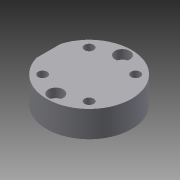
# Autodesk Inventor part: 02-2-0.125-FO1_BM_heads_left-bif
Saved by Autodesk Inventor 2014 SP2 (Build 180246200, 246)
## iProperties
Created: 2020-02-04
Part Number: 02-2-0.125-FO1_BM_heads_left-bif
Material: Generic
Catalog Web Link: www.cadenas.de
Description: FO1 Basic Model Heads_left-Bimba FLAT-1
Vendor: BIMBA
Document SubType Name: Modeling
Designer: psadmin
Manufacturer: BIMBA
Mass: 4.51427 g
Surface Area: 26.3958 cm^2
Volume: 4.51427 cm^3
Density: 1 g/cm^3
Appearance: PSOLRGB-211-211-211
Category: PARTsolutions
Company: BIMBA
Title: 02-2-0.125-FO1_BM_heads_left-bif
Author: Cadenas PARTsolutions
Comments: Bimba FLAT-1
PSOL_IDENT_0: {$CADENAS_DATA\23d-libs\bimba\bimba_brand\bimba_imperial\bimba_full_line\flat_cylinders\fo1\fo1_basi
PSOL_IDENT_1: c_model_heads_left.prj},279 {VTYP=3D},{NB=02-2-0.125-FO1_BM_heads_left-bif},{LINA=02-2-0.125-FO1_BM_
PSOL_IDENT_2: heads_left-bif},{NN=FO1 Basic Model Heads_left},{DATE=22.01.2020 09:06:03},{GEOMDATE=10.10.2019 07:1
PSOL_IDENT_3: 7:43},{VERSION=},{LINEID=10},{WBVAR=MNT,LRR,ER,RTX,HD,STPT1,STPT2,STPT3,STPT4,PP,MRS,RL1},{WBNUMERIC=
PSOL_IDENT_4: RL1}  {NB=02-2-0.125-FO1_BM_heads_left-bif},{LINA=02-2-0.125-FO1_BM_heads_left-bif},{KT=DUMMY},{PN=0
PSOL_IDENT_5: 2-2-0.125-FO1_BM_heads_left},{BORE=0.56250000},{BOREPN=02},{MNT=},{MNTALG='','Standard Counterbored
PSOL_IDENT_6: Mounting Holes','1','Pivot Mount','1N','Pivot Mount 90 Deg. from Standard','2','[2] Trunnion Mount','
PSOL_IDENT_7: 3R','Threaded Mounting Holes, Rear','4R','Screw Clearance Holes, Rear','6','F Series Interchange, Co
PSOL_IDENT_8: unterbored, Rear [6]' ,'7R','F Series Interchange, Threaded, Rear [7R]'},{LRR=2},{ER=},{RTX=},{RTXAL
PSOL_IDENT_9: G='', 'Standard', 'CFT', 'Coarse Female Thread', 'CMT'  , 'Male Rod Thread (Coarse)','MT', 'Male Rod
PSOL_IDENT_10: End (Fine)', 'NT'  , 'Non-Threaded Rod'},{HD=},{STPT1=},{STPT2=},{STPT3=},{STPT4=},{PP=},{MRS=},{PP
PSOL_IDENT_11: ALG='','Standard'},{A=1.11300000},{C=0.87500000},{AR=0.88000000},{DD=2.00000000},{D=0.11200000},{CPI
PSOL_IDENT_12: L=0.12850000},{DC=0.17900000},{DCP=0.12000000},{DCD=0.85500000},{ES=0.16400000},{EC=0.00000000},{ED=
PSOL_IDENT_13: 0.46000000},{F=0.25000000},{H=0.22000000},{J=0.344},{J1=0.34400000},{K=0.172},{K1=0.17200000},{K2=0.
PSOL_IDENT_14: 27000000},{L=0.19000000},{LDP=0.20000000},{LP=0.16000000},{LPDP=0.28000000},{TD=0.61000000},{TDDP=0.
PSOL_IDENT_15: 10000},{LSF=0.31250000},{LSFDP=0.02300000},{AA=0.06000000},{AB=0.75000000},{AC=0.38000000},{AD=0.500
PSOL_IDENT_16: 00000},{AD1=UNF},{AE=0.49750000},{AF=0.31000000},{M=0.00000000},{N=0.00000000},{P=0.00000000},{Q=0.1
PSOL_IDENT_17: 9000000},{QQ=0.252},{R=0.11200000},{S=0.37500000},{T=0.19000000},{U=0.25000000},{W=0.75000000},{X=0.
PSOL_IDENT_18: 18500000},{Y=0.63000000},{Z=0.19000000},{A13=0.11200000},{A14=0.16600000},{ANGLE=45.00000000},{JY=0.
PSOL_IDENT_19: 344},{JH=0.344},{PANGLE=0},{ANGLE1=45},{ANGLE11=45.00000000},{D11=0.1285},{CONX=0.12000000},{CONY=0.
PSOL_IDENT_20: 12000000},{G=0.29000000},{HH=0.54000000},{RD=0.24000000},{HDADD1=0.13000000},{HDADD=0},{GW=0.0775},{
PSOL_IDENT_21: GD=0.4215},{GR=0.0315},{PW=0.0620},{PD=0.4975},{PR=0.0150},{RL1=0.12500},{CS=0.86400},{DS=0.12850},{
PSOL_IDENT_22: DCS=0.20000},{DCSP=0.15000},{C4=0.89000},{CD=0.87500},{C6=0.87500},{D6=0.15400},{DC6=0.23600},{DC6P=
PSOL_IDENT_23: 0.14800},{C7=0.87500},{R7=0.13800},{RC=0.86400},{RT=0.112},{RCB=0.12000},{RCD=0.10000},{PB1=0.375},{
PSOL_IDENT_24: PB2=0.1905},{JB=0},{AP=1.1150},{PCB=0.2000},{PCD=0.1360},{PCBD=0.120},{ALPH=60},{BDIA=0.650},{BD=0.0
PSOL_IDENT_25: 27},{MNTRG=},{JS=0.09375},{TL=0.375},{NANG=45.0}
NN: FO1 Basic Model Heads_left
NT: Bimba FLAT-1
NB: 02-2-0.125-FO1_BM_heads_left-bif
NBSYN: $PN.-bif
LINA: 02-2-0.125-FO1_BM_heads_left-bif
PN: 02-2-0.125-FO1_BM_heads_left
BORE: 0
BOREPN: 02
MNT: Standard Counterbored Mounting Holes
LRR: 2
ER: Single Rod
RTX: Standard
HD: Standard Rear Head
STPT1: Without T1
STPT2: Without T2
STPT3: Without T3
STPT4: Without T4
PP: Standard
MRS: Without -Z
A: 1.113
C: 0.875
AR: 0.88
DD: 2
D: 0.112
CPIL: 0.1285
DC: 0.179
DCP: 0.12
DCD: 0.855
ES: 0.164
EC: 0
ED: 0.46
F: 0.25
H: 0.22
J1: 0.344
K1: 0.172
K2: 0.27
L: 0.19
LDP: 0.2
LP: 0.16
LPDP: 0.28
TD: 0.61
TDDP: 0.1
LSF: 0.3125
LSFDP: 0.023
AA: 0.06
AB: 0.75
AC: 0.38
AD: 0.5
AD1: UNF
AE: 0.4975
AF: 0.31
M: 0
N: 0
P: 0
Q: 0.19
QQ: 0.252
R: 0.112
S: 0.375
T: 0.19
U: 0.25
W: 0.75
X: 0.185
Y: 0.63
Z: 0.19
A13: 0.112
A14: 0.166
ANGLE: 45
ANGLE11: 45
CONX: 0.12
CONY: 0.12
G: 0.29
HH: 0.54
RD: 0.24
HDADD1: 0.13
GW: 0.0775
GD: 0.4215
GR: 0.0315
PW: 0.062
PD: 0.4975
PR: 0.015
RL1: 0.125
CS: 0.864
DS: 0.1285
DCS: 0.2
DCSP: 0.15
C4: 0.89
C6: 0.875
D6: 0.154
DC6: 0.236
DC6P: 0.148
C7: 0.875
R7: 0.138
RC: 0.864
RT: 0.112
RCB: 0.12
RCD: 0.1
PB1: 0.375
PB2: 0.1905
AP: 1.115
PCB: 0.2
PCD: 0.136
PCBD: 0.12
BDIA: 0.65
BD: 0.027
JS: 0.09375
TL: 0.375
NANG: 45
SUPPLIER: BIMBA
ARTICLENO: 02-2-0.125-FO1_BM_heads_left-bif
BOMINFO: 02-2-0.125-FO1_BM_heads_left-bif
CREATOR: CADENAS GmbH
Autodesk Inventor part; units mm, degrees
sketch "Sketch_1" plane through (0, 0, 0) normal (0, 0, 1) x (1, 0, 0)
  line L0 (0, 0) -> (0, 8.7376)
  line L1 (0, 8.7376) -> (14.1351, 8.7376)
  line L2 (14.1351, 8.7376) -> (14.1351, 0)
  line L3 (14.1351, 0) -> (0, 0)
  line L4 (0, 0) -> (0, 8.7376)
  constraints: 10 end point
revolve "Revolution1" add sketch "Sketch_1" angle 360 about axis through (0, 0, 0) along (0, -1, 0)
sketch "Sketch_63" plane through (0, 0, 0) normal (0, 1, 0) x (-1, 0, 0)
  line L0 (20.6184, 14.1351) -> (13.5509, 14.1351)
  line L1 (13.5509, 14.1351) -> (13.5509, -14.1351)
  line L2 (13.5509, -14.1351) -> (20.6184, -14.1351)
  line L3 (20.6184, -14.1351) -> (20.6184, 14.1351)
  constraints: 8 end point
extrude "Extrusion1" cut sketch "Sketch_63" along normal blind 8.7376
sketch "Sketch_37" plane through (0, 0, 0) normal (0, 0, 1) x (1, 0, 0)
  line L0 (-5.8778, 4.3688) -> (-14.1351, 4.3688)
  line L1 (-14.1351, 4.3688) -> (-14.1351, 8.3376)
  line L2 (-14.1351, 8.3376) -> (-13.5509, 8.3376)
  line L3 (-13.5509, 8.3376) -> (-13.5509, 6.7818)
  line L4 (-13.5509, 6.7818) -> (-13.1216, 6.3525)
  line L5 (-13.1216, 6.3525) -> (-7.0231, 6.3525)
  line L6 (-7.0231, 6.3525) -> (-5.8778, 4.3688)
  line L7 (-5.8778, 4.3688) -> (-14.1351, 4.3688)
  constraints: 16 end point
revolve "Revolution2" cut sketch "Sketch_37" angle 360 about axis through (-5.8778, 4.3688, 0) along (1, 0, 0)
thread "Thread1" size "10-32 UNF" class "2B" standard "ANSI Unified Screw Threads" length 4.6507
sketch "Sketch4" plane through (0, 0, 0) normal (0, -1, 0) x (1, 0, 0)
  point P0 (0, 0)
hole "Hole1" at (0, 0, 0) direction (0, 1, 0) diameter 15.494 depth 2.54
sketch "Sketch5" plane through (0, 8.7376, 0) normal (0, 1, 0) x (1, 0, 0)
  point P0 (0, -11.1125)
hole "Hole2" at (0, 8.7376, 11.1125) direction (0, -1, 0) diameter 3.2639 depth 8.7376 counterbore diameter 4.953 counterbore depth 3.048
sketch "Sketch6" plane through (0, 8.7376, 0) normal (0, 1, 0) x (1, 0, 0)
  point P0 (0, 11.1125)
hole "Hole3" at (0, 8.7376, -11.1125) direction (0, -1, 0) diameter 3.2639 depth 8.7376 counterbore diameter 4.953 counterbore depth 3.048
sketch "Sketch7" plane through (0, 8.7376, 0) normal (0, 1, 0) x (1, 0, 0)
  point P0 (-7.7589, -7.7589)
hole "Hole4" at (-7.7589, 8.7376, 7.7589) direction (0, -1, 0) diameter 2.1565 depth 8.7376 counterbore diameter 3.048 counterbore depth 2.54 thread size "4-40 UNC" class "2B" standard "ANSI Unified Screw Threads"
pattern_linear "Rectangular Pattern1" count 2 spacing 15.5179 along (1, 0, 0) count 2 spacing 15.5179 along (0, 0, -1) of "Hole4"
ref_plane "a1_XY" through (0, 8.7376, -14.1351) normal (0, 1, 0) x (1, 0, 0)
ref_plane "a1_YZ" through (0, 8.7376, -14.1351) normal (1, 0, 0) x (0, 0, -1)
ref_plane "a1_ZX" through (0, 8.7376, -14.1351) normal (0, 0, -1) x (0, 1, 0)
ref_plane "a2_XY" through (0, 8.7376, 14.1351) normal (0, 1, 0) x (1, 0, 0)
ref_plane "a2_YZ" through (0, 8.7376, 14.1351) normal (1, 0, 0) x (0, 0, -1)
ref_plane "a2_ZX" through (0, 8.7376, 14.1351) normal (0, 0, -1) x (0, 1, 0)
ref_plane "ar3_XY" through (-7.9026, 2.54, 7.9026) normal (0, 1, 0) x (1, 0, 0)
ref_plane "ar3_YZ" through (-7.9026, 2.54, 7.9026) normal (1, 0, 0) x (0, 0, -1)
ref_plane "ar3_ZX" through (-7.9026, 2.54, 7.9026) normal (0, 0, -1) x (0, 1, 0)
ref_plane "ar4_XY" through (7.9026, 2.54, 7.9026) normal (0, 1, 0) x (1, 0, 0)
ref_plane "ar4_YZ" through (7.9026, 2.54, 7.9026) normal (1, 0, 0) x (0, 0, -1)
ref_plane "ar4_ZX" through (7.9026, 2.54, 7.9026) normal (0, 0, -1) x (0, 1, 0)
ref_plane "ar5_XY" through (7.9026, 2.54, -7.9026) normal (0, 1, 0) x (1, 0, 0)
ref_plane "ar5_YZ" through (7.9026, 2.54, -7.9026) normal (1, 0, 0) x (0, 0, -1)
ref_plane "ar5_ZX" through (7.9026, 2.54, -7.9026) normal (0, 0, -1) x (0, 1, 0)
ref_plane "ar6_XY" through (-7.9026, 2.54, -7.9026) normal (0, 1, 0) x (1, 0, 0)
ref_plane "ar6_YZ" through (-7.9026, 2.54, -7.9026) normal (1, 0, 0) x (0, 0, -1)
ref_plane "ar6_ZX" through (-7.9026, 2.54, -7.9026) normal (0, 0, -1) x (0, 1, 0)
ref_plane "b1_XY" through (0, 8.7376, 0) normal (0, 1, 0) x (1, 0, 0)
ref_plane "b1_YZ" through (0, 8.7376, 0) normal (1, 0, 0) x (0, 0, -1)
ref_plane "b1_ZX" through (0, 8.7376, 0) normal (0, 0, -1) x (0, 1, 0)
ref_plane "j_XY" through (0, 0, 0) normal (0, 1, 0) x (1, 0, 0)
ref_plane "j_YZ" through (0, 0, 0) normal (1, 0, 0) x (0, 0, -1)
ref_plane "j_ZX" through (0, 0, 0) normal (0, 0, -1) x (0, 1, 0)
ref_plane "k1_XY" through (-13.5509, 4.3688, 0) normal (0, 0, 1) x (1, 0, 0)
ref_plane "k1_YZ" through (-13.5509, 4.3688, 0) normal (1, 0, 0) x (0, 1, 0)
ref_plane "k1_ZX" through (-13.5509, 4.3688, 0) normal (0, 1, 0) x (0, 0, 1)
ref_plane "k2_XY" through (-13.5509, 8.7376, 0) normal (0, 0, 1) x (1, 0, 0)
ref_plane "k2_YZ" through (-13.5509, 8.7376, 0) normal (1, 0, 0) x (0, 1, 0)
ref_plane "k2_ZX" through (-13.5509, 8.7376, 0) normal (0, 1, 0) x (0, 0, 1)
ref_plane "l1_XY" through (-13.5509, 6.7818, 0) normal (0, 0, 1) x (1, 0, 0)
ref_plane "l1_YZ" through (-13.5509, 6.7818, 0) normal (1, 0, 0) x (0, 1, 0)
ref_plane "l1_ZX" through (-13.5509, 6.7818, 0) normal (0, 1, 0) x (0, 0, 1)
ref_plane "l2_XY" through (-13.5509, 1.9558, 0) normal (0, 0, 1) x (1, 0, 0)
ref_plane "l2_YZ" through (-13.5509, 1.9558, 0) normal (1, 0, 0) x (0, 1, 0)
ref_plane "l2_ZX" through (-13.5509, 1.9558, 0) normal (0, 1, 0) x (0, 0, 1)
ref_plane "po1_XY" through (10.9728, 0, 0) normal (0, 1, 0) x (1, 0, 0)
ref_plane "po1_YZ" through (10.9728, 0, 0) normal (1, 0, 0) x (0, 0, -1)
ref_plane "po1_ZX" through (10.9728, 0, 0) normal (0, 0, -1) x (0, 1, 0)
ref_plane "po2_XY" through (-5.4864, 0, -9.5027) normal (0, 1, 0) x (1, 0, 0)
ref_plane "po2_YZ" through (-5.4864, 0, -9.5027) normal (1, 0, 0) x (0, 0, -1)
ref_plane "po2_ZX" through (-5.4864, 0, -9.5027) normal (0, 0, -1) x (0, 1, 0)
ref_plane "po3_XY" through (-5.4864, 0, 9.5027) normal (0, 1, 0) x (1, 0, 0)
ref_plane "po3_YZ" through (-5.4864, 0, 9.5027) normal (1, 0, 0) x (0, 0, -1)
ref_plane "po3_ZX" through (-5.4864, 0, 9.5027) normal (0, 0, -1) x (0, 1, 0)
ref_plane "r7_XY" through (-1.7526, 8.7376, -11.1125) normal (0, 1, 0) x (1, 0, 0)
ref_plane "r7_YZ" through (-1.7526, 8.7376, -11.1125) normal (1, 0, 0) x (0, 0, -1)
ref_plane "r7_ZX" through (-1.7526, 8.7376, -11.1125) normal (0, 0, -1) x (0, 1, 0)
ref_plane "r71_XY" through (0, 8.7376, 11.1125) normal (0, 1, 0) x (1, 0, 0)
ref_plane "r71_YZ" through (0, 8.7376, 11.1125) normal (1, 0, 0) x (0, 0, -1)
ref_plane "r71_ZX" through (0, 8.7376, 11.1125) normal (0, 0, -1) x (0, 1, 0)
ref_plane "r72_XY" through (1.7526, 8.7376, -11.1125) normal (0, 1, 0) x (1, 0, 0)
ref_plane "r72_YZ" through (1.7526, 8.7376, -11.1125) normal (1, 0, 0) x (0, 0, -1)
ref_plane "r72_ZX" through (1.7526, 8.7376, -11.1125) normal (0, 0, -1) x (0, 1, 0)
ref_plane "r73_XY" through (0, 8.7376, -11.1125) normal (0, 1, 0) x (1, 0, 0)
ref_plane "r73_YZ" through (0, 8.7376, -11.1125) normal (1, 0, 0) x (0, 0, -1)
ref_plane "r73_ZX" through (0, 8.7376, -11.1125) normal (0, 0, -1) x (0, 1, 0)
ref_plane "rg_XY" through (0, 8.7376, 0) normal (0, 1, 0) x (1, 0, 0)
ref_plane "rg_YZ" through (0, 8.7376, 0) normal (1, 0, 0) x (0, 0, -1)
ref_plane "rg_ZX" through (0, 8.7376, 0) normal (0, 0, -1) x (0, 1, 0)
ref_plane "rh_XY" through (0, 8.7376, 0) normal (0, 1, 0) x (1, 0, 0)
ref_plane "rh_YZ" through (0, 8.7376, 0) normal (1, 0, 0) x (0, 0, -1)
ref_plane "rh_ZX" through (0, 8.7376, 0) normal (0, 0, -1) x (0, 1, 0)
ref_plane "rs_1_XY" through (0, 10.5156, -11.1125) normal (0, 1, 0) x (1, 0, 0)
ref_plane "rs_1_YZ" through (0, 10.5156, -11.1125) normal (1, 0, 0) x (0, 0, -1)
ref_plane "rs_1_ZX" through (0, 10.5156, -11.1125) normal (0, 0, -1) x (0, 1, 0)
ref_plane "rs_2_XY" through (-11.1125, 10.5156, 0) normal (0, 1, 0) x (1, 0, 0)
ref_plane "rs_2_YZ" through (-11.1125, 10.5156, 0) normal (1, 0, 0) x (0, 0, -1)
ref_plane "rs_2_ZX" through (-11.1125, 10.5156, 0) normal (0, 0, -1) x (0, 1, 0)
ref_plane "rs_3_XY" through (0, 10.5156, 11.1125) normal (0, 1, 0) x (1, 0, 0)
ref_plane "rs_3_YZ" through (0, 10.5156, 11.1125) normal (1, 0, 0) x (0, 0, -1)
ref_plane "rs_3_ZX" through (0, 10.5156, 11.1125) normal (0, 0, -1) x (0, 1, 0)
ref_plane "rs_4_XY" through (11.1125, 10.5156, 0) normal (0, 1, 0) x (1, 0, 0)
ref_plane "rs_4_YZ" through (11.1125, 10.5156, 0) normal (1, 0, 0) x (0, 0, -1)
ref_plane "rs_4_ZX" through (11.1125, 10.5156, 0) normal (0, 0, -1) x (0, 1, 0)
ref_plane "sc1_XY" through (10.9728, 4.9276, 0) normal (0, 1, 0) x (1, 0, 0)
ref_plane "sc1_YZ" through (10.9728, 4.9276, 0) normal (1, 0, 0) x (0, 0, -1)
ref_plane "sc1_ZX" through (10.9728, 4.9276, 0) normal (0, 0, -1) x (0, 1, 0)
ref_plane "sc2_XY" through (-5.4864, 4.9276, -9.5027) normal (0, 1, 0) x (1, 0, 0)
ref_plane "sc2_YZ" through (-5.4864, 4.9276, -9.5027) normal (1, 0, 0) x (0, 0, -1)
ref_plane "sc2_ZX" through (-5.4864, 4.9276, -9.5027) normal (0, 0, -1) x (0, 1, 0)
ref_plane "sc3_XY" through (-5.4864, 4.9276, 9.5027) normal (0, 1, 0) x (1, 0, 0)
ref_plane "sc3_YZ" through (-5.4864, 4.9276, 9.5027) normal (1, 0, 0) x (0, 0, -1)
ref_plane "sc3_ZX" through (-5.4864, 4.9276, 9.5027) normal (0, 0, -1) x (0, 1, 0)
ref_plane "to_dummy_XY" through (0, 8.7376, 0) normal (0, 1, 0) x (1, 0, 0)
ref_plane "to_dummy_YZ" through (0, 8.7376, 0) normal (1, 0, 0) x (0, 0, -1)
ref_plane "to_dummy_ZX" through (0, 8.7376, 0) normal (0, 0, -1) x (0, 1, 0)
ref_plane "to_nut_XY" through (0, 10.2616, 0) normal (0, 1, 0) x (1, 0, 0)
ref_plane "to_nut_YZ" through (0, 10.2616, 0) normal (1, 0, 0) x (0, 0, -1)
ref_plane "to_nut_ZX" through (0, 10.2616, 0) normal (0, 0, -1) x (0, 1, 0)
ref_plane "to_rod_XY" through (0, 8.7376, 0) normal (0, 1, 0) x (1, 0, 0)
ref_plane "to_rod_YZ" through (0, 8.7376, 0) normal (1, 0, 0) x (0, 0, -1)
ref_plane "to_rod_ZX" through (0, 8.7376, 0) normal (0, 0, -1) x (0, 1, 0)
ref_plane "to_tube_XY" through (0, 2.54, 0) normal (0, 1, 0) x (1, 0, 0)
ref_plane "to_tube_YZ" through (0, 2.54, 0) normal (1, 0, 0) x (0, 0, -1)
ref_plane "to_tube_ZX" through (0, 2.54, 0) normal (0, 0, -1) x (0, 1, 0)
ref_plane "to_wiper_XY" through (0, 8.7376, 0) normal (0, 1, 0) x (1, 0, 0)
ref_plane "to_wiper_YZ" through (0, 8.7376, 0) normal (1, 0, 0) x (0, 0, -1)
ref_plane "to_wiper_ZX" through (0, 8.7376, 0) normal (0, 0, -1) x (0, 1, 0)
ref_plane "track1_XY" through (-7.7851, 0, 0) normal (0, 1, 0) x (1, 0, 0)
ref_plane "track1_YZ" through (-7.7851, 0, 0) normal (1, 0, 0) x (0, 0, -1)
ref_plane "track1_ZX" through (-7.7851, 0, 0) normal (0, 0, -1) x (0, 1, 0)
ref_plane "track2_XY" through (0, 0, -7.7851) normal (0, 1, 0) x (1, 0, 0)
ref_plane "track2_YZ" through (0, 0, -7.7851) normal (1, 0, 0) x (0, 0, -1)
ref_plane "track2_ZX" through (0, 0, -7.7851) normal (0, 0, -1) x (0, 1, 0)
ref_plane "track3_XY" through (7.7851, 0, 0) normal (0, 1, 0) x (1, 0, 0)
ref_plane "track3_YZ" through (7.7851, 0, 0) normal (1, 0, 0) x (0, 0, -1)
ref_plane "track3_ZX" through (7.7851, 0, 0) normal (0, 0, -1) x (0, 1, 0)
ref_plane "track4_XY" through (0, 0, 7.7851) normal (0, 1, 0) x (1, 0, 0)
ref_plane "track4_YZ" through (0, 0, 7.7851) normal (1, 0, 0) x (0, 0, -1)
ref_plane "track4_ZX" through (0, 0, 7.7851) normal (0, 0, -1) x (0, 1, 0)
body "Solid1"
